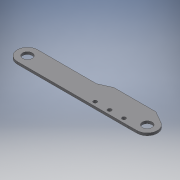
# Autodesk Inventor part: rinnku
Saved by Autodesk Inventor 2018 (Build 220112000, 112)
## iProperties
Created: 2016-08-23
Part Number: rinnku
Material: GFRP
Document SubType Name: Modeling
Designer: hiro
Density: 1.75 g/cm^3
Appearance: 滑らか - 淡い灰色
Mass: 6.14531 g
Surface Area: 43.3352 cm^2
Volume: 3.5116 cm^3
Author: hiro
Autodesk Inventor part; units mm, degrees
ref_plane "YZ Plane" through (0, 0, 0) normal (1, 0, 0) x (0, 1, 0)
ref_plane "XZ Plane" through (0, 0, 0) normal (0, 1, 0) x (-1, 0, 0)
ref_plane "XY Plane" through (0, 0, 0) normal (0, 0, 1) x (1, 0, 0)
sketch "スケッチ1" plane through (0, 0, 0) normal (0, 0, 1) x (1, 0, 0)
  line L0 (-50, 0) -> (50, 0) construction
  circle A0 centre (-50, 0) radius 4.05
  circle A1 centre (50, 0) radius 4.05
  line L1 (-50, 8.5) -> (43, 8.5)
  line L2 (-50, -8.5) -> (43, -8.5)
  arc A2 (-50, 8.5) -> (-50, -8.5) centre (-50, 0) ccw
  line L3 (43, -8.5) -> (50.119, -8.3992)
  line L4 (43, 8.5) -> (50.119, 8.3992)
  arc A3 (50.119, -8.3992) -> (50.119, 8.3992) centre (50, 0) ccw
  line L5 (9, -7.5) -> (38, -7.5) construction
  line L6 (38, -7.5) -> (38, -2.5) construction
  line L7 (38, -2.5) -> (9, -2.5) construction
  line L8 (9, -2.5) -> (9, -7.5) construction
  line L9 (9, -5) -> (38, -5) construction
  circle A4 centre (23.5, -5) radius 1.55
  circle A5 centre (11.5, -5) radius 1.55
  circle A6 centre (35.5, -5) radius 1.55
  line L10 (23.5, -5) -> (23.5, -2.5) construction
  line L11 (44.1615, 13) -> (9.1615, 13)
  line L12 (9.1615, 13) -> (-0.8385, 8.5)
  line L13 (44.1615, 13) -> (54.1615, 7.2967)
  point P0 (0, 0)
  point P1 (0, 0)
  point P2 (52.0517, 8.5)
  dimension "d0" = 100
  dimension "d1" = 8.1
  dimension "d2" = 8.5
  dimension "d8" = 8.1
  dimension "d9" = 7
  dimension "d10" = 8.4
  dimension "d12" = 5
  dimension "d13" = 29
  dimension "d14" = 3.1
  dimension "d15" = 2.5
  dimension "d17" = 13
  dimension "d19" = 10
  dimension "d20" = 35
  dimension "d25" = 12
  dimension "d26" = 10
  dimension "d34" = 1
  constraints: 28 end point, 7 centre point, 5 horizontal, 5 midpoint, 5 point on circle, 5 point on line, 5 tangent, 4 coincident, 2 equal radius, 2 parallel, 1 perpendicular, 1 symmetric about line, 1 vertical alignment
  measures "d0" distance of L0.start L0.end
  measures "d1" diameter of A0
  measures "d2" radius of A2
  measures "d8" diameter of A1
  measures "d9" horizontal distance of L1.end L0.end
  measures "d10" radius of A3
  measures "d12" distance of L7.end L5.start
  measures "d13" distance of L6.end L7.end
  measures "d14" diameter of A4
  measures "d15" distance from line of L8 A5.centre
  measures "d17" distance from line of L0.end L11
  measures "d19" horizontal distance of L12.end L11.end
  measures "d20" distance of L11.start L11.end
  measures "d25" distance from line of L0.end L6
  measures "d26" horizontal distance of L11.start L13.end
  measures "d34" distance between parallel lines of L2 L5
extrude "押し出し1" add sketch "スケッチ1" along normal blind 2
fillet "フィレット1" radius 2 3 edges at (-0.8385, 8.5, 1) (9.1615, 13, 1) (44.1615, 13, 1)
equation "\"d8\" = d1"
equation "\"d19\" = d18"
equation "\"d26\" = d19"
equation "\"d18\" = 10"
